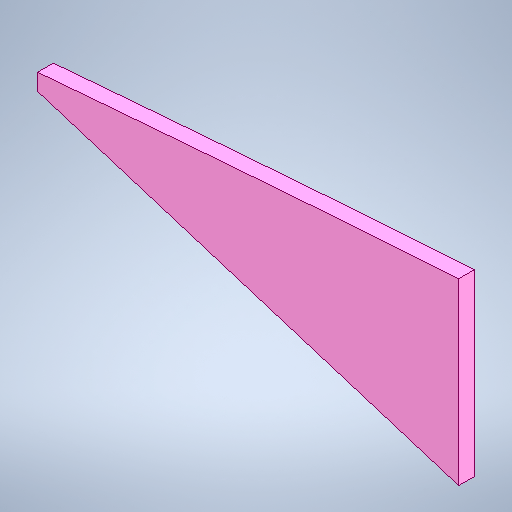
# Autodesk Inventor part: Part2
Saved by Autodesk Inventor 2025.3 (Build 293356030, 356C)
## iProperties
Created: 2025-07-04
Part Number: Part2
Material: Generic
Document SubType Name: Modeling
Designer: steve
Density: 1 g/cm^3
Appearance: Default(1)
Author: steve
Autodesk Inventor part; units mm, degrees
ref_plane "YZ Plane" through (0, 0, 0) normal (1, 0, 0) x (0, 1, 0)
ref_plane "XZ Plane" through (0, 0, 0) normal (0, 1, 0) x (-1, 0, 0)
ref_plane "XY Plane" through (0, 0, 0) normal (0, 0, 1) x (1, 0, 0)
sketch "Sketch1" plane through (0, 0, 0) normal (0, 0, 1) x (1, 0, 0)
  line L0 (0, 0) -> (80, 0)
  line L1 (80, 0) -> (80, -28)
  line L2 (0, 0) -> (0, -3.14)
  line L3 (0, -3.14) -> (80, -28)
  line L4 (150.2892, -0.1489) -> (150.2892, 5.4009)
  line L5 (230.2892, -0.1489) -> (230.2892, 1.7609)
  spline S0 degree 2 poles (80, 6.0264) (44.0347, 3.6882) (0, 0) knots 1.817648 1.817648 1.817648 2 2 2
  line L6 (44.0347, 3.6882) -> (0, 0) construction
  line L7 (80, 0) -> (80, 6.0264)
  line L8 (80, 6.0264) -> (44.0347, 3.6882) construction
  point P0 (56.2982, -5.2891)
  point P1 (80, 6.0264)
  dimension "d1" = 28
  dimension "d4" = 3.14
  dimension "d16" = 80
  constraints: 14 end point, 2 vertical, 1 horizontal, 3 other
  measures "d1" distance of L0.end L1.end
  measures "d4" distance of L0.start L2.end
  measures "d16" distance of L0.start L0.end
extrude "Extrusion1" add sketch "Sketch1" along normal blind 3
body "Solid1"
